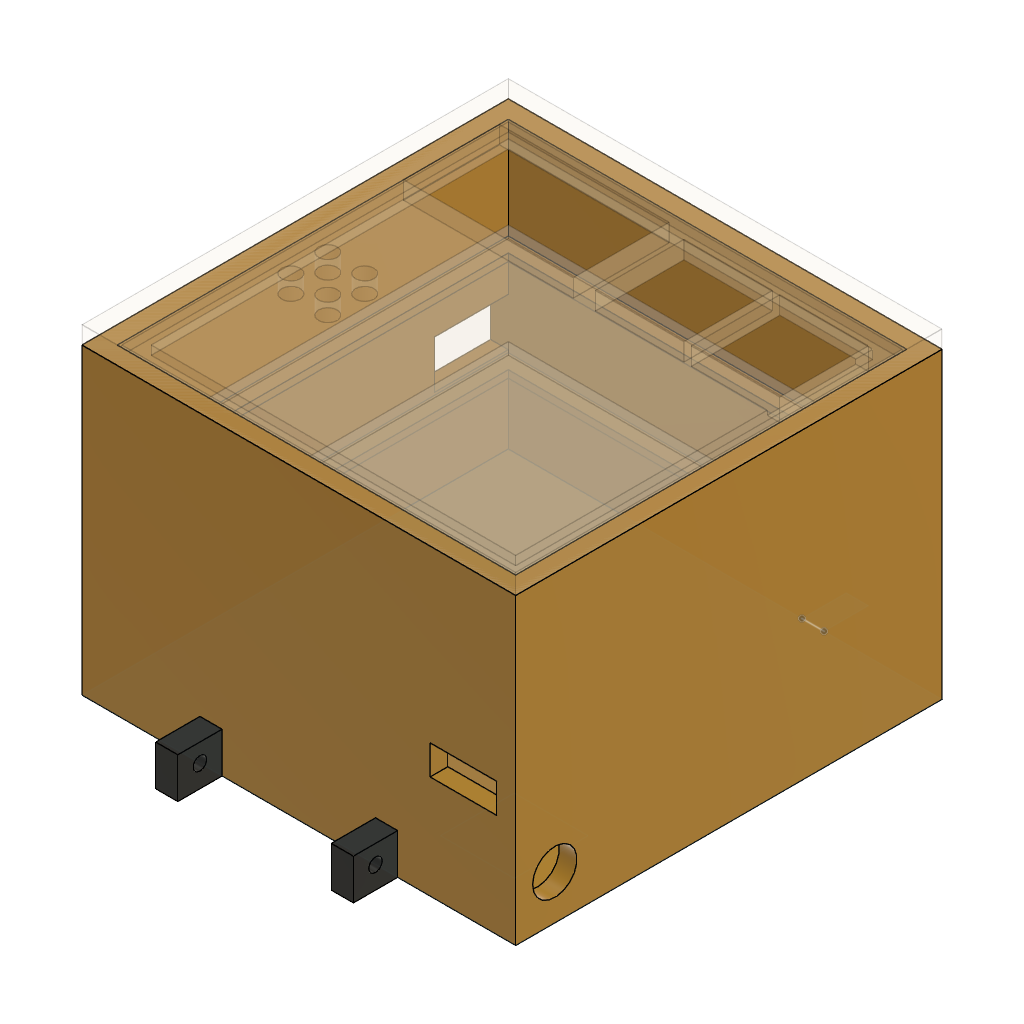
3DCase (Autodesk Fusion 360 design; units mm, degrees)
part number: 2026-10-04-11-01-38-182
part number: 2026-10-04-11-13-21-206
part number: 2026-10-04-11-13-29-976
part number: 2026-10-04-11-13-39-671
Autodesk Fusion 360 part; units mm, degrees
sketch "Sketch1" plane through (0, 0, 0) normal (0, 1, 0) x (1, 0, 0) in component "Shelf"
sketch "Sketch1 (2)" plane through (0, 0, 0) normal (0, 1, 0) x (1, 0, 0) in component "Base"
  line L0 (0, 0) -> (58.8, 0)
  line L1 (58.8, 0) -> (58.8, -57.8)
  line L2 (58.8, -57.8) -> (0, -57.8)
  line L3 (0, -57.8) -> (0, 0)
  constraint horizontal L0
  constraint vertical L1
  constraint horizontal L2
  constraint vertical L3
  constraint coincident L0.start L3.end
sketch "Sketch2" plane through (0, 0, 57.8) normal (0, 0, 1) x (-1, 0, 0) in component "Base"
sketch "Sketch3" plane through (0, 0, 0) normal (0, 0, 1) x (1, 0, 0) in component "Base"
  line L0 (0, 0) -> (-58.8, 0)
  line L1 (-58.8, 0) -> (-58.8, -57.8)
  line L2 (-58.8, -57.8) -> (0, -57.8)
  line L3 (0, -57.8) -> (0, 0)
  dimension "d12" = 58.8
  dimension "d13" = 57.8
  constraint coincident L0.start L3.end
  constraint horizontal L0
  constraint perpendicular L0 L1
  constraint perpendicular L1 L2
  constraint perpendicular L0 L3
  measures "d12" distance of L0.start L0.end
  measures "d13" distance of L0.end L1.end
extrude "Extrude2" add sketch "Sketch3" along normal blind 41.1 makes body 1 in component "Base"
sketch "Sketch4" plane through (0, 0, 41.1) normal (0, 0, 1) x (-1, 0, 0) in component "Base"
  line L0 (0, 57.8) -> (0, 0)
  line L1 (0, 0) -> (58.8, 0)
  line L2 (58.8, 0) -> (58.8, 57.8)
  line L3 (58.8, 57.8) -> (0, 57.8)
  line L4 (0, 0) -> (2.4, 0)
  line L5 (2.4, 0) -> (2.4, 2.4)
  line L6 (2.4, 2.4) -> (0, 2.4)
  line L7 (0, 2.4) -> (0, 0)
  line L8 (2.4, 2.4) -> (56.4, 2.4)
  line L9 (56.4, 2.4) -> (56.4, 55.4)
  line L10 (56.4, 55.4) -> (2.4, 55.4)
  line L11 (2.4, 55.4) -> (2.4, 2.4)
  dimension "d16" = 2.4
  dimension "d17" = 2.4
  dimension "d18" = 54
  dimension "d19" = 53
  constraint horizontal L4
  constraint vertical L5
  constraint horizontal L6
  constraint vertical L7
  constraint coincident L0.end L1.start
  constraint horizontal L8
  constraint vertical L9
  constraint horizontal L10
  constraint vertical L11
  measures "d16" distance of L0.end L4.end
  measures "d17" distance of L0.end L6.end
  measures "d18" distance of L5.end L8.end
  measures "d19" distance of L5.end L10.end
extrude "Extrude3" cut sketch "Sketch4" against normal blind 38.7 contours L8 L9 L10 L11 bodies 1 in component "Base"
ref_plane "WorkPlane3" through (-29.4, -28.9, 10.3) normal (0, 0, -1) x (-1, 0, 0) in component "Base"
sketch "Sketch6" plane through (0, 0, 10.3) normal (0, 0, -1) x (-1, 0, 0) in component "Base"
ref_plane "WorkPlane4" through (-29.4, -28.9, 12.7) normal (0, 0, 1) x (1, 0, 0) in component "Base"
sketch "Sketch7" plane through (0, 0, 12.7) normal (0, 0, 1) x (1, 0, 0) in component "Base"
ref_plane "WorkPlane5" through (-29.4, -28.9, 12.7) normal (0, 0, 1) x (1, 0, 0) in component "Base"
sketch "Sketch8" plane through (0, 0, 12.7) normal (0, 0, 1) x (1, 0, 0) in component "Base"
  line L0 (-56.4, -2.4) -> (-2.4, -2.4)
  line L1 (-2.4, -2.4) -> (-2.4, -55.4)
  line L2 (-2.4, -55.4) -> (-56.4, -55.4)
  line L3 (-56.4, -55.4) -> (-56.4, -2.4)
  line L4 (-56.4, -2.4) -> (-54.4, -2.4)
  line L5 (-56.4, -4.4) -> (-56.4, -2.4)
  line L6 (-54.4, -4.4) -> (-4.4, -4.4)
  line L7 (-4.4, -4.4) -> (-4.4, -53.4)
  line L8 (-4.4, -53.4) -> (-54.4, -53.4)
  line L9 (-54.4, -53.4) -> (-54.4, -4.4)
  dimension "d36" = 2
  dimension "d37" = 2
  dimension "d38" = 50
  dimension "d39" = 49
  constraint horizontal L0
  constraint vertical L1
  constraint horizontal L2
  constraint vertical L3
  constraint horizontal L4
  constraint vertical L5
  constraint horizontal L6
  constraint vertical L7
  constraint horizontal L8
  constraint vertical L9
  measures "d36" distance of L0.start L4.end
  measures "d37" distance of L0.start L5.start
  measures "d38" distance of L6.start L6.end
  measures "d39" distance of L6.start L8.end
extrude "Extrude4" add sketch "Sketch8" along normal blind 1 bodies 1 in component "Base"
sketch "Sketch9" plane through (-58.8, 0, 0) normal (-1, 0, 0) x (0, -1, 0) in component "Base"
  line L0 (0, 0) -> (57.8, 0)
  line L1 (57.8, 0) -> (57.8, 41.1)
  line L2 (57.8, 41.1) -> (0, 41.1)
  line L3 (0, 41.1) -> (0, 0)
  line L4 (23, 2.9) -> (33, 2.9)
  line L5 (33, 2.9) -> (33, 7.9)
  line L6 (33, 7.9) -> (23, 7.9)
  line L7 (23, 7.9) -> (23, 2.9)
  dimension "d46" = 10
  dimension "d47" = 5
  constraint horizontal L4
  constraint vertical L5
  constraint horizontal L6
  constraint vertical L7
  measures "d46" distance of L4.start L4.end
  measures "d47" distance of L4.start L6.end
extrude "Extrude5" cut sketch "Sketch9" against normal blind 2.9 contours L4 L5 L6 L7 bodies 1 in component "Base"
ref_plane "WorkPlane7" through (-29.4, -28.9, 27.4) normal (0, 0, -1) x (-1, 0, 0) in component "Base"
sketch "Sketch10" plane through (0, 0, 27.4) normal (0, 0, -1) x (-1, 0, 0) in component "Base"
  line L0 (2.4, -55.4) -> (56.4, -55.4)
  line L1 (56.4, -55.4) -> (56.4, -2.4)
  line L2 (56.4, -2.4) -> (2.4, -2.4)
  line L3 (2.4, -2.4) -> (2.4, -55.4)
  line L4 (4.4, -53.4) -> (54.4, -53.4)
  line L5 (54.4, -53.4) -> (54.4, -4.4)
  line L6 (54.4, -4.4) -> (4.4, -4.4)
  line L7 (4.4, -4.4) -> (4.4, -53.4)
  constraint horizontal L0
  constraint vertical L1
  constraint horizontal L2
  constraint vertical L3
  constraint horizontal L4
  constraint vertical L5
  constraint horizontal L6
  constraint vertical L7
extrude "Extrude6" add sketch "Sketch10" along normal blind 1 bodies 1 in component "Base"
sketch "Sketch11" plane through (-58.8, 0, 0) normal (-1, 0, 0) x (0, -1, 0) in component "Base"
  line L0 (33, 2.9) -> (23, 2.9)
  line L1 (23, 2.9) -> (23, 7.9)
  line L2 (23, 7.9) -> (33, 7.9)
  line L3 (33, 7.9) -> (33, 2.9)
  line L4 (0, 0) -> (57.8, 0)
  line L5 (57.8, 0) -> (57.8, 41.1)
  line L6 (57.8, 41.1) -> (0, 41.1)
  line L7 (0, 41.1) -> (0, 0)
  line L8 (23, 14) -> (33, 14)
  line L9 (33, 14) -> (33, 20.5)
  line L10 (33, 20.5) -> (23, 20.5)
  line L11 (23, 20.5) -> (23, 14)
  dimension "d55" = 6.5
  constraint horizontal L8
  constraint vertical L9
  constraint horizontal L10
  constraint vertical L11
  measures "d55" distance of L8.start L10.end
extrude "Extrude7" cut sketch "Sketch11" against normal blind 2.4 contours L8 L9 L10 L11 bodies 1 in component "Base"
sketch "Sketch12" plane through (-58.8, 0, 0) normal (-1, 0, 0) x (0, -1, 0) in component "Base"
  line L0 (33, 14) -> (23, 14)
  line L1 (23, 14) -> (23, 20.5)
  line L2 (23, 20.5) -> (33, 20.5)
  line L3 (33, 20.5) -> (33, 14)
  line L4 (33, 2.9) -> (23, 2.9)
  line L5 (23, 2.9) -> (23, 7.9)
  line L6 (23, 7.9) -> (33, 7.9)
  line L7 (33, 7.9) -> (33, 2.9)
  line L8 (0, 0) -> (57.8, 0)
  line L9 (57.8, 0) -> (57.8, 41.1)
  line L10 (57.8, 41.1) -> (0, 41.1)
  line L11 (0, 41.1) -> (0, 0)
  line L12 (2.4, 20.55) -> (12.4, 20.55)
  line L13 (12.4, 20.55) -> (12.4, 14.05)
  line L14 (12.4, 14.05) -> (2.4, 14.05)
  line L15 (2.4, 14.05) -> (2.4, 20.55)
  dimension "d60" = 10
  dimension "d61" = 6.5
  constraint horizontal L12
  constraint vertical L13
  constraint horizontal L14
  constraint vertical L15
  measures "d60" distance of L12.start L12.end
  measures "d61" distance of L12.start L14.end
extrude "Extrude8" cut sketch "Sketch12" against normal blind 2.4 contours L12 L13 L14 L15 bodies 1 in component "Base"
sketch "Sketch13" plane through (-58.8, 0, 0) normal (-1, 0, 0) x (0, -1, 0) in component "Base"
  line L0 (12.4, 20.55) -> (12.4, 14.05)
  line L1 (12.4, 14.05) -> (2.4, 14.05)
  line L2 (2.4, 14.05) -> (2.4, 20.55)
  line L3 (2.4, 20.55) -> (12.4, 20.55)
  line L4 (33, 14) -> (23, 14)
  line L5 (23, 14) -> (23, 20.5)
  line L6 (23, 20.5) -> (33, 20.5)
  line L7 (33, 20.5) -> (33, 14)
  line L8 (33, 2.9) -> (23, 2.9)
  line L9 (23, 2.9) -> (23, 7.9)
  line L10 (23, 7.9) -> (33, 7.9)
  line L11 (33, 7.9) -> (33, 2.9)
  line L12 (0, 0) -> (57.8, 0)
  line L13 (57.8, 0) -> (57.8, 41.1)
  line L14 (57.8, 41.1) -> (0, 41.1)
  line L15 (0, 41.1) -> (0, 0)
  line L16 (57.8, 7.9) -> (55.4, 7.9)
  line L17 (55.4, 7.9) -> (55.4, 5.5)
  line L18 (55.4, 5.5) -> (57.8, 5.5)
  line L19 (57.8, 5.5) -> (57.8, 7.9)
  line L20 (55.4, 7.9) -> (45.4, 7.9)
  line L21 (45.4, 7.9) -> (45.4, 2.9)
  line L22 (45.4, 2.9) -> (55.4, 2.9)
  line L23 (55.4, 2.9) -> (55.4, 7.9)
  dimension "d64" = 2.4
  dimension "d65" = 2.4
  dimension "d66" = 10
  dimension "d67" = 5
  constraint horizontal L16
  constraint vertical L17
  constraint horizontal L18
  constraint vertical L19
  constraint coincident L13 L16.start
  constraint horizontal L20
  constraint vertical L21
  constraint horizontal L22
  constraint vertical L23
  measures "d64" distance of L16.start L16.end
  measures "d65" distance of L16.start L18.end
  measures "d66" distance of L16.end L20.end
  measures "d67" distance of L16.end L22.end
extrude "Extrude9" cut sketch "Sketch13" against normal blind 2.4 contours L17 L20 L21 L22 L23 bodies 1 in component "Base"
sketch "Sketch14" plane through (-58.8, 0, 0) normal (-1, 0, 0) x (0, -1, 0) in component "Base"
  line L0 (45.4, 7.9) -> (55.4, 7.9)
  line L1 (55.4, 7.9) -> (55.4, 2.9)
  line L2 (55.4, 2.9) -> (45.4, 2.9)
  line L3 (45.4, 2.9) -> (45.4, 7.9)
  line L4 (12.4, 20.55) -> (12.4, 14.05)
  line L5 (12.4, 14.05) -> (2.4, 14.05)
  line L6 (2.4, 14.05) -> (2.4, 20.55)
  line L7 (2.4, 20.55) -> (12.4, 20.55)
  line L8 (33, 14) -> (23, 14)
  line L9 (33, 20.5) -> (33, 14)
  line L10 (33, 2.9) -> (23, 2.9)
  line L11 (23, 2.9) -> (23, 7.9)
  line L12 (23, 7.9) -> (33, 7.9)
  line L13 (33, 7.9) -> (33, 2.9)
  line L14 (0, 0) -> (57.8, 0)
  line L15 (57.8, 0) -> (57.8, 41.1)
  line L16 (57.8, 41.1) -> (0, 41.1)
  line L17 (0, 41.1) -> (0, 0)
  line L18 (33, 20.5) -> (23, 20.5)
  line L19 (23, 20.5) -> (23, 14)
  line L20 (23, 14) -> (33, 14)
  line L21 (33, 14) -> (33, 20.5)
  constraint horizontal L18
  constraint vertical L19
  constraint horizontal L20
  constraint vertical L21
  constraint coincident L8.end L19.end
  constraint coincident L9.start L18.start
extrude "Extrude10" add sketch "Sketch14" against normal blind 2.4 contours L8 L9 L18 L19 L20 L21 bodies 1 in component "Base"
sketch "Sketch15" plane through (-58.8, 0, 0) normal (-1, 0, 0) x (0, -1, 0) in component "Base"
  line L0 (45.4, 7.9) -> (55.4, 7.9)
  line L1 (55.4, 7.9) -> (55.4, 2.9)
  line L2 (55.4, 2.9) -> (45.4, 2.9)
  line L3 (45.4, 2.9) -> (45.4, 7.9)
  line L4 (12.4, 20.55) -> (12.4, 14.05)
  line L5 (12.4, 14.05) -> (2.4, 14.05)
  line L6 (2.4, 14.05) -> (2.4, 20.55)
  line L7 (2.4, 20.55) -> (12.4, 20.55)
  line L8 (33, 2.9) -> (23, 2.9)
  line L9 (23, 2.9) -> (23, 7.9)
  line L10 (0, 0) -> (57.8, 0)
  line L11 (57.8, 0) -> (57.8, 41.1)
  line L12 (57.8, 41.1) -> (0, 41.1)
  line L13 (0, 41.1) -> (0, 0)
  line L14 (23, 7.9) -> (33, 7.9)
  line L15 (33, 7.9) -> (33, 2.9)
  line L16 (33, 2.9) -> (23, 2.9)
  line L17 (23, 2.9) -> (23, 7.9)
  constraint horizontal L14
  constraint vertical L15
  constraint horizontal L16
  constraint vertical L17
  constraint coincident L8.start L15.end
  constraint coincident L9.end L14.start
extrude "Extrude11" add sketch "Sketch15" against normal blind 2.4 contours L8 L9 L14 L15 L16 L17 bodies 1 in component "Base"
sketch "Sketch16" plane through (0, 0, 0) normal (1, 0, 0) x (0, 1, 0) in component "Base"
  line L0 (-57.8, 0) -> (0, 0)
  line L1 (0, 0) -> (0, 41.1)
  line L2 (0, 41.1) -> (-57.8, 41.1)
  line L3 (-57.8, 41.1) -> (-57.8, 0)
  circle A0 centre (-52.5, 6) radius 3
  dimension "d76" = 6
  measures "d76" diameter of A0
extrude "Extrude12" cut sketch "Sketch16" against normal blind 2.4 contours A0 bodies 1 in component "Base"
sketch "Sketch17" plane through (0, -57.8, 0) normal (0, -1, 0) x (1, 0, 0) in component "Base"
  line L0 (-58.8, 0) -> (0, 0)
  line L1 (0, 0) -> (0, 41.1)
  line L2 (0, 41.1) -> (-58.8, 41.1)
  line L3 (-58.8, 41.1) -> (-58.8, 0)
  line L4 (-2.6, 14) -> (-11.6, 14)
  line L5 (-11.6, 14) -> (-11.6, 18)
  line L6 (-11.6, 18) -> (-2.6, 18)
  line L7 (-2.6, 18) -> (-2.6, 14)
  dimension "d80" = 9
  dimension "d81" = 4
  constraint horizontal L4
  constraint vertical L5
  constraint horizontal L6
  constraint vertical L7
  measures "d80" distance of L4.start L4.end
  measures "d81" distance of L4.start L6.end
extrude "Extrude13" cut sketch "Sketch17" against normal blind 2.4 contours L4 L5 L6 L7 bodies 1 in component "Base"
sketch "Sketch18" plane through (0, 0, 2.4) normal (0, 0, 1) x (-1, 0, 0) in component "Base"
  line L0 (2.4, 55.4) -> (2.4, 2.4)
  line L1 (2.4, 2.4) -> (56.4, 2.4)
  line L2 (56.4, 2.4) -> (56.4, 55.4)
  line L3 (56.4, 55.4) -> (2.4, 55.4)
  line L4 (8, 50) -> (18, 50)
  line L5 (18, 50) -> (18, 40)
  line L6 (18, 40) -> (8, 40)
  line L7 (8, 40) -> (8, 50)
  dimension "d84" = 10
  dimension "d85" = 10
  constraint horizontal L4
  constraint vertical L5
  constraint horizontal L6
  constraint vertical L7
  measures "d84" distance of L4.start L4.end
  measures "d85" distance of L4.start L6.end
extrude "Extrude14" cut sketch "Sketch18" against normal blind 2.4 contours L4 L5 L6 L7 bodies 1 in component "Base"
sketch "Sketch19" plane through (0, -57.8, 0) normal (0, -1, 0) x (1, 0, 0) in component "Base"
  line L0 (-11.6, 14) -> (-11.6, 18)
  line L1 (-11.6, 18) -> (-2.6, 18)
  line L2 (-2.6, 18) -> (-2.6, 14)
  line L3 (-2.6, 14) -> (-11.6, 14)
  line L4 (-58.8, 0) -> (0, 0)
  line L5 (0, 0) -> (0, 41.1)
  line L6 (0, 41.1) -> (-58.8, 41.1)
  line L7 (-58.8, 41.1) -> (-58.8, 0)
  line L8 (-16, 0) -> (-19, 0)
  line L9 (-19, 0) -> (-19, 5.5)
  line L10 (-19, 5.5) -> (-16, 5.5)
  line L11 (-16, 5.5) -> (-16, 0)
  dimension "d88" = 3
  dimension "d89" = 5.5
  constraint horizontal L8
  constraint vertical L9
  constraint horizontal L10
  constraint vertical L11
  measures "d88" distance of L8.start L8.end
  measures "d89" distance of L8.start L10.end
extrude "Extrude15" add sketch "Sketch19" along normal blind 6 separate body contours L4 L8 L9 L10 L11 makes body 2 in component "Base"
sketch "Sketch20" plane through (0, -57.8, 0) normal (0, -1, 0) x (1, 0, 0) in component "Base"
  line L0 (-11.6, 14) -> (-11.6, 18)
  line L1 (-11.6, 18) -> (-2.6, 18)
  line L2 (-2.6, 18) -> (-2.6, 14)
  line L3 (-2.6, 14) -> (-11.6, 14)
  line L4 (-58.8, 0) -> (0, 0)
  line L5 (0, 0) -> (0, 41.1)
  line L6 (0, 41.1) -> (-58.8, 41.1)
  line L7 (-58.8, 41.1) -> (-58.8, 0)
  line L8 (-42.8, 0) -> (-39.8, 0)
  line L9 (-39.8, 0) -> (-39.8, 5.5)
  line L10 (-39.8, 5.5) -> (-42.8, 5.5)
  line L11 (-42.8, 5.5) -> (-42.8, 0)
  dimension "d92" = 16
  dimension "d94" = 3
  constraint horizontal L8
  constraint vertical L9
  constraint horizontal L10
  constraint vertical L11
  measures "d92" distance of L4.start L8.start
  measures "d94" distance of L8.start L8.end
extrude "Extrude16" add sketch "Sketch20" along normal blind 6 separate body contours L4 L8 L9 L10 L11 makes body 3 in component "Base"
sketch "Sketch21" plane through (0, 0, 0) normal (0, 1, 0) x (-1, 0, 0) in component "Base"
  line L0 (0, 0) -> (58.8, 0)
  line L1 (58.8, 0) -> (58.8, 41.1)
  line L2 (58.8, 41.1) -> (0, 41.1)
  line L3 (0, 41.1) -> (0, 0)
  line L4 (16, 0) -> (19, 0)
  line L5 (19, 0) -> (19, 5.5)
  line L6 (19, 5.5) -> (16, 5.5)
  line L7 (16, 5.5) -> (16, 0)
  dimension "d97" = 16
  dimension "d99" = 3
  dimension "d100" = 5.5
  constraint horizontal L4
  constraint vertical L5
  constraint horizontal L6
  constraint vertical L7
  measures "d97" distance of L0.start L4.start
  measures "d99" distance of L4.start L4.end
  measures "d100" distance of L4.start L6.end
extrude "Extrude17" add sketch "Sketch21" along normal blind 6 contours L0 L4 L5 L6 L7 bodies 1 in component "Base"
sketch "Sketch22" plane through (0, 0, 0) normal (0, 1, 0) x (-1, 0, 0) in component "Base"
  line L0 (19, 5.5) -> (19, 0)
  line L1 (19, 0) -> (58.8, 0)
  line L2 (58.8, 0) -> (58.8, 41.1)
  line L3 (58.8, 41.1) -> (0, 41.1)
  line L4 (0, 41.1) -> (0, 0)
  line L5 (0, 0) -> (16, 0)
  line L6 (16, 0) -> (16, 5.5)
  line L7 (16, 5.5) -> (19, 5.5)
  line L8 (42.8, 0) -> (39.8, 0)
  line L9 (39.8, 0) -> (39.8, 5.5)
  line L10 (39.8, 5.5) -> (42.8, 5.5)
  line L11 (42.8, 5.5) -> (42.8, 0)
  dimension "d103" = 16
  dimension "d105" = 3
  dimension "d106" = 5.5
  constraint horizontal L8
  constraint vertical L9
  constraint horizontal L10
  constraint vertical L11
  measures "d103" distance of L1.end L8.start
  measures "d105" distance of L8.start L8.end
  measures "d106" distance of L8.start L10.end
extrude "Extrude18" add sketch "Sketch22" along normal blind 6 separate body contours L1 L8 L9 L10 L11 makes body 4 in component "Base"
sketch "Sketch23" plane through (-42.8, 0, 0) normal (-1, 0, 0) x (0, -1, 0) in component "Base"
  line L0 (57.8, 5.5) -> (57.8, 0)
  line L1 (57.8, 0) -> (63.8, 0)
  line L2 (63.8, 0) -> (63.8, 5.5)
  line L3 (63.8, 5.5) -> (57.8, 5.5)
  circle A0 centre (60.8, 3) radius 0.9
  dimension "d111" = 1.8
  measures "d111" diameter of A0
extrude "Extrude19" cut sketch "Sketch23" against normal blind 3 contours A0 bodies 3 in component "Base"
sketch "Sketch24" plane through (-16, 0, 0) normal (1, 0, 0) x (0, 1, 0) in component "Base"
  line L0 (-57.8, 0) -> (-57.8, 5.5)
  line L1 (-57.8, 5.5) -> (-63.8, 5.5)
  line L2 (-63.8, 5.5) -> (-63.8, 0)
  line L3 (-63.8, 0) -> (-57.8, 0)
  circle A0 centre (3, 3) radius 0.9
  dimension "d116" = 1.8
  measures "d116" diameter of A0
extrude "Extrude20" cut sketch "Sketch24" against normal blind 3 contours A0 bodies 1 in component "Base"
sketch "Sketch25" plane through (-16, 0, 0) normal (1, 0, 0) x (0, 1, 0) in component "Base"
  line L0 (-57.8, 0) -> (-57.8, 5.5)
  line L1 (-57.8, 5.5) -> (-63.8, 5.5)
  line L2 (-63.8, 5.5) -> (-63.8, 0)
  line L3 (-63.8, 0) -> (-57.8, 0)
  circle A0 centre (-60.8, 3) radius 0.9
  dimension "d121" = 1.8
  measures "d121" diameter of A0
extrude "Extrude21" cut sketch "Sketch25" against normal blind 3 contours A0 bodies 2 in component "Base"
sketch "Sketch26" plane through (-42.8, 0, 0) normal (-1, 0, 0) x (0, -1, 0) in component "Base"
  line L0 (0, 0) -> (0, 5.5)
  line L1 (0, 5.5) -> (-6, 5.5)
  line L2 (-6, 5.5) -> (-6, 0)
  line L3 (-6, 0) -> (0, 0)
  circle A0 centre (-3, 3) radius 0.9
  dimension "d126" = 1.8
  measures "d126" diameter of A0
extrude "Extrude22" cut sketch "Sketch26" against normal blind 3 contours A0 bodies 4 in component "Base"
sketch "Sketch1 (3)" plane through (0, 0, 41.1) normal (0, 0, 1) x (-1, 0, 0) in component "Lid"
  line L0 (56.4, 2.4) -> (2.4, 2.4)
  line L1 (2.4, 2.4) -> (2.4, 55.4)
  line L2 (2.4, 55.4) -> (56.4, 55.4)
  line L3 (56.4, 55.4) -> (56.4, 2.4)
  line L4 (0, 57.8) -> (0, 0)
  line L5 (0, 0) -> (58.8, 0)
  line L6 (58.8, 0) -> (58.8, 57.8)
  line L7 (58.8, 57.8) -> (0, 57.8)
  line L8 (0, 57.8) -> (58.8, 57.8)
  line L9 (58.8, 57.8) -> (58.8, 0)
  line L10 (58.8, 0) -> (0, 0)
  line L11 (0, 0) -> (0, 57.8)
  constraint horizontal L8
  constraint vertical L9
  constraint horizontal L10
  constraint vertical L11
  constraint coincident L5.end L6.start
  constraint coincident L4.start L7.end
extrude "Extrude1" add sketch "Sketch1 (3)" along normal blind 2.4 separate body contours L0 L1 L2 L3 | L4 L5 L6 L7 L8 L9 L10 L11 makes body 5 in component "Lid"
sketch "Sketch2 (2)" plane through (0, 0, 43.5) normal (0, 0, 1) x (-1, 0, 0) in component "Lid"
  line L0 (0, 0) -> (58.8, 0)
  line L1 (58.8, 0) -> (58.8, 57.8)
  line L2 (58.8, 57.8) -> (0, 57.8)
  line L3 (0, 57.8) -> (0, 0)
  line L4 (2.7, 2.7) -> (56.1, 2.7)
  line L5 (56.1, 2.7) -> (56.1, 55.1)
  line L6 (56.1, 55.1) -> (2.7, 55.1)
  line L7 (2.7, 55.1) -> (2.7, 2.7)
  dimension "d133" = 53.4
  dimension "d134" = 52.4
  constraint horizontal L4
  constraint vertical L5
  constraint horizontal L6
  constraint vertical L7
  measures "d133" distance of L4.start L4.end
  measures "d134" distance of L4.start L6.end
extrude "Extrude2'" add sketch "Sketch2 (2)" against normal blind 1.2 bodies 5 in component "Lid"
sketch "Sketch3 (2)" plane through (0, 0, 43.5) normal (0, 0, 1) x (-1, 0, 0) in component "Lid"
  line L0 (0, 0) -> (58.8, 0)
  line L1 (58.8, 0) -> (58.8, 57.8)
  line L2 (58.8, 57.8) -> (0, 57.8)
  line L3 (0, 57.8) -> (0, 0)
  line L4 (2, 55.8) -> (54.4, 55.8)
  line L5 (54.4, 55.8) -> (54.4, 2.4)
  line L6 (54.4, 2.4) -> (2, 2.4)
  line L7 (2, 2.4) -> (2, 55.8)
  dimension "d139" = 52.4
  dimension "d140" = 53.4
  constraint horizontal L4
  constraint vertical L5
  constraint horizontal L6
  constraint vertical L7
  measures "d139" distance of L4.start L4.end
  measures "d140" distance of L4.start L6.end
extrude "Extrude3'" add sketch "Sketch3 (2)" against normal blind 1.2 bodies 5 in component "Lid"
sketch "Sketch4 (2)" plane through (0, 0, 43.5) normal (0, 0, 1) x (-1, 0, 0) in component "Lid"
  line L0 (0, 0) -> (58.8, 0)
  line L1 (58.8, 0) -> (58.8, 57.8)
  line L2 (58.8, 57.8) -> (0, 57.8)
  line L3 (0, 57.8) -> (0, 0)
  line L4 (2.7, 55.1) -> (56.1, 55.1)
  line L5 (56.1, 55.1) -> (56.1, 2.7)
  line L6 (56.1, 2.7) -> (2.7, 2.7)
  line L7 (2.7, 2.7) -> (2.7, 55.1)
  line L8 (4.7, 4.7) -> (4.7, 53.1)
  line L9 (4.7, 53.1) -> (54.1, 53.1)
  line L10 (54.1, 53.1) -> (54.1, 4.7)
  line L11 (54.1, 4.7) -> (4.7, 4.7)
  dimension "d145" = 53.4
  dimension "d146" = 52.4
  dimension "d147" = 2
  constraint horizontal L4
  constraint vertical L5
  constraint horizontal L6
  constraint vertical L7
  measures "d145" distance of L4.start L4.end
  measures "d146" distance of L4.start L6.end
extrude "Extrude4'" add sketch "Sketch4 (2)" against normal blind 1.2 contours L4 L5 L6 L7 bodies 5 in component "Lid"
sketch "Sketch5" plane through (0, 0, 41.1) normal (0, 0, -1) x (1, 0, 0) in component "Lid"
  line L0 (-58.8, 0) -> (0, 0)
  line L1 (0, 0) -> (0, 57.8)
  line L2 (0, 57.8) -> (-58.8, 57.8)
  line L3 (-58.8, 57.8) -> (-58.8, 0)
  line L4 (-2.7, 2.7) -> (-56.1, 2.7)
  line L5 (-56.1, 2.7) -> (-56.1, 55.1)
  line L6 (-56.1, 55.1) -> (-2.7, 55.1)
  line L7 (-2.7, 55.1) -> (-2.7, 2.7)
  line L8 (-4.7, 4.7) -> (-54.1, 4.7)
  line L9 (-54.1, 4.7) -> (-54.1, 53.1)
  line L10 (-54.1, 53.1) -> (-4.7, 53.1)
  line L11 (-4.7, 53.1) -> (-4.7, 4.7)
  dimension "d152" = 53.4
  dimension "d153" = 52.4
  dimension "d154" = 2
  constraint horizontal L4
  constraint vertical L5
  constraint horizontal L6
  constraint vertical L7
  measures "d152" distance of L4.start L4.end
  measures "d153" distance of L4.start L6.end
extrude "Extrude5'" add sketch "Sketch5" along normal blind 1.2 contours L4 L5 L6 L7 bodies 5 in component "Lid"
sketch "Sketch6 (2)" plane through (0, 0, 43.5) normal (0, 0, 1) x (-1, 0, 0) in component "Lid"
  line L0 (0, 0) -> (58.8, 0)
  line L1 (58.8, 0) -> (58.8, 57.8)
  line L2 (58.8, 57.8) -> (0, 57.8)
  line L3 (0, 57.8) -> (0, 0)
  line L4 (54, 6) -> (31, 6)
  line L5 (31, 6) -> (31, 19)
  line L6 (31, 19) -> (54, 19)
  line L7 (54, 19) -> (54, 6)
  line L8 (3, 7) -> (15, 7)
  line L9 (15, 7) -> (15, 19)
  line L10 (15, 19) -> (3, 19)
  line L11 (3, 19) -> (3, 7)
  line L12 (16, 7) -> (28, 7)
  line L13 (28, 7) -> (28, 19)
  line L14 (28, 19) -> (16, 19)
  line L15 (16, 19) -> (16, 7)
  circle A0 centre (50.6355, 32.6313) radius 1.25
  circle A1 centre (50.6355, 37.6313) radius 1.25
  circle A2 centre (45.6355, 37.6313) radius 1.25
  circle A3 centre (45.6355, 32.6313) radius 1.25
  dimension "d159" = 23
  dimension "d160" = 13
  dimension "d163" = 12
  dimension "d164" = 12
  dimension "d165" = 12
  dimension "d166" = 12
  dimension "d173" = 2.5
  dimension "d180" = 2.5
  dimension "d181" = 2.5
  dimension "d182" = 2.5
  constraint horizontal L4
  constraint vertical L5
  constraint horizontal L6
  constraint vertical L7
  constraint horizontal L8
  constraint vertical L9
  constraint horizontal L10
  constraint vertical L11
  constraint horizontal L12
  constraint vertical L13
  constraint horizontal L14
  constraint vertical L15
  measures "d159" distance of L4.start L4.end
  measures "d160" distance of L4.start L6.end
  measures "d163" distance of L8.start L8.end
  measures "d164" distance of L8.start L10.end
  measures "d165" distance of L12.start L12.end
  measures "d166" distance of L12.start L14.end
  measures "d173" diameter of A0
  measures "d180" diameter of A1
  measures "d181" diameter of A2
  measures "d182" diameter of A3
extrude "Extrude6'" cut sketch "Sketch6 (2)" against normal blind 3 contours L4 L5 L6 L7 | L8 L9 L10 L11 | L12 L13 L14 L15 | A0 | A1 | A2 | A3 bodies 5 in component "Lid"
ref_plane "WorkPlane1" through (-29.4, -25.9, 13.9) normal (0, 0, -1) x (-1, 0, 0) in component "Shelf"
sketch "Sketch2 (3)" plane through (0, 0, 13.9) normal (0, 0, -1) x (-1, 0, 0) in component "Shelf"
  line L0 (2.7, -55.1) -> (56.1, -55.1)
  line L1 (56.1, -55.1) -> (56.1, -2.7)
  line L2 (56.1, -2.7) -> (2.7, -2.7)
  line L3 (2.7, -2.7) -> (2.7, -55.1)
  line L4 (56.1, -10.5) -> (56.1, -2.7)
  line L5 (8.6, -10.5) -> (13.1, -10.5)
  line L6 (13.1, -10.5) -> (13.1, -22.5)
  line L7 (13.1, -22.5) -> (8.6, -22.5)
  line L8 (8.6, -22.5) -> (8.6, -10.5)
  dimension "d195" = 4.5
  dimension "d196" = 12
  constraint horizontal L0
  constraint vertical L1
  constraint horizontal L2
  constraint vertical L3
  constraint vertical L4
  constraint horizontal L5
  constraint vertical L6
  constraint horizontal L7
  constraint vertical L8
  measures "d195" distance of L5.start L5.end
  measures "d196" distance of L5.start L7.end
extrude "Extrude1'" add sketch "Sketch2 (3)" against normal blind 1.6 separate body makes body 6 in component "Shelf"
copy_body "CopyPasteBodies1" bodies 6 makes body 7 in component "Shelf"
move_body "Move1" bodies 7 to x (1, 0, 0) y (0, 1, 0) z (0, 0, 1) at (0, 0, 13.5) in component "Shelf"
move_body "Move2" bodies 6 to x (1, 0, 0) y (0, 1, 0) z (0, 0, 1) at (0, 0, -0.2) in component "Shelf"
sketch "Sketch27" plane through (0, 0, 0) normal (0, 0, -1) x (1, 0, 0) in component "Base"
  line L0 (-18, 40) -> (-18, 50)
  line L1 (-18, 50) -> (-8, 50)
  line L2 (-8, 50) -> (-8, 40)
  line L3 (-8, 40) -> (-18, 40)
  line L4 (0, 0) -> (0, 57.8)
  line L5 (0, 57.8) -> (-58.8, 57.8)
  line L6 (-58.8, 57.8) -> (-58.8, 0)
  line L7 (-58.8, 0) -> (-19, 0)
  line L8 (-19, 0) -> (-19, -6)
  line L9 (-19, -6) -> (-16, -6)
  line L10 (-16, -6) -> (-16, 0)
  line L11 (-16, 0) -> (0, 0)
  line L12 (-16, 0) -> (-19, 0)
  constraint coincident L10.end L11.start
  constraint coincident L7.end L8.start
component "Base" placed x (1, 0, 0) y (0, 1, 0) z (0, 0, 1) at (0, 0, 0)
component "Lid" placed x (1, 0, 0) y (0, 1, 0) z (0, 0, 1) at (0, 0, 0)
component "Shelf" placed x (1, 0, 0) y (0, 1, 0) z (0, 0, 1) at (0, 0, 0)
equation "in_x = 54 mm"
equation "in_y = 53 mm"
equation "wall = 2.4 mm"
equation "floor_t = 2.4 mm"
equation "z_top = 41.1 mm"
